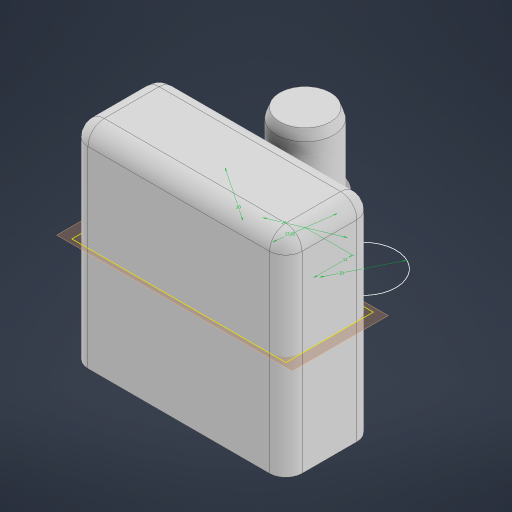
# Autodesk Inventor part: batteriehalter
Saved by Autodesk Inventor 2023 (Build 270158000, 158)
## iProperties
Created: 2023-05-28
Part Number: batteriehalter
Material: Generic
Document SubType Name: Modeling
Designer: bananenbrot
Density: 1 g/cm^3
Appearance: Default
Author: bananenbrot
Autodesk Inventor part; units mm, degrees
ref_plane "YZ Plane" through (0, 0, 0) normal (1, 0, 0) x (0, 1, 0)
ref_plane "XZ Plane" through (0, 0, 0) normal (0, 1, 0) x (-1, 0, 0)
ref_plane "XY Plane" through (0, 0, 0) normal (0, 0, 1) x (1, 0, 0)
sketch "Sketch1" plane through (0, 0, 0) normal (0, 1, 0) x (-1, 0, 0)
  line L0 (3.8011, 12.3974) -> (-62.0989, 12.3974)
  line L1 (-62.0989, 12.3974) -> (-62.0989, -14.5026)
  line L2 (-62.0989, -14.5026) -> (3.8011, -14.5026)
  line L3 (3.8011, -14.5026) -> (3.8011, 12.3974)
  line L4 (2.6011, 11.1974) -> (-60.8989, 11.1974)
  line L5 (-60.8989, 11.1974) -> (-60.8989, -13.3026)
  line L6 (-60.8989, -13.3026) -> (2.6011, -13.3026)
  line L7 (2.6011, -13.3026) -> (2.6011, 11.1974)
  point P0 (0, 0)
  dimension "d0" = 26.9
  dimension "d1" = 65.9
  dimension "d2" = 1.2
  dimension "d3" = 24.5
  dimension "d4" = 63.5
  constraints: 16 end point, 4 parallel, 2 perpendicular, 1 horizontal, 3 other
  measures "d0" distance of L2.end L0.start
  measures "d1" distance of L0.start L0.end
  measures "d2" distance between parallel lines of L3 L7
  measures "d3" distance of L6.end L4.start
  measures "d4" distance of L5.end L6.end
extrude "Extrusion1" add sketch "Sketch1" along normal blind 1.2 contours L3 L2 L1 L0 | L7 L6 L5 L4
extrude "Extrusion2" add sketch "Sketch1" against normal blind 63
fillet "Fillet1" radius 5 8 edges at (29.1489, 0, 11.1974) (-2.6011, -31.5, 11.1974) (-2.6011, 0, -1.0526) (29.1489, 0, -13.3026) (60.8989, 0, -1.0526) (60.8989, -31.5, -13.3026) (-2.6011, -31.5, -13.3026) (60.8989, -31.5, 11.1974)
ref_plane "Work Plane1" through (0, -30.9, 0) normal (0, 1, 0) x (1, 0, 0)
sketch "Sketch3" plane through (0, -30.9, 0) normal (0, 1, 0) x (1, 0, 0)
  arc A0 (2.3989, 13.3026) -> (-2.6011, 8.3026) centre (2.3989, 8.3026) ccw projected
  line L0 (-2.6011, 8.3026) -> (-2.6011, -6.1974) projected
  arc A1 (-2.6011, -6.1974) -> (2.3989, -11.1974) centre (2.3989, -6.1974) ccw projected
  line L1 (2.3989, -11.1974) -> (55.8989, -11.1974) projected
  arc A2 (55.8989, -11.1974) -> (60.8989, -6.1974) centre (55.8989, -6.1974) ccw projected
  line L2 (60.8989, -6.1974) -> (60.8989, 8.3026) projected
  arc A3 (60.8989, 8.3026) -> (55.8989, 13.3026) centre (55.8989, 8.3026) ccw projected
  line L3 (55.8989, 13.3026) -> (2.3989, 13.3026) projected
  line L4 (62.0989, -12.3974) -> (-3.8011, -12.3974) projected
  line L5 (-3.8011, -12.3974) -> (-3.8011, 14.5026) projected
  line L6 (-3.8011, 14.5026) -> (62.0989, 14.5026) projected
  line L7 (62.0989, 14.5026) -> (62.0989, -12.3974) projected
  circle A4 centre (29.1489, 26.5026) radius 8.825
  circle A5 centre (29.1489, 26.5026) radius 10
  circle A6 centre (9.2492, 24.5026) radius 10
  circle A7 centre (49.0487, 24.5026) radius 10
  point P0 (0, 0)
  point P1 (29.1489, 14.5026)
  point P2 (49.0487, 14.5026)
  point P3 (39.0988, 25.5026)
  point P4 (19.199, 25.5026)
  point P5 (9.2492, 14.5026)
  dimension "d10" = 17.65
  dimension "d11" = 20
  dimension "d12" = 12
  dimension "d13" = 20
  dimension "d14" = 20
  constraints: 4 centre point, 4 tangent, 1 coincident, 1 midpoint, 1 vertical alignment
  measures "d10" diameter of A4
  measures "d11" diameter of A5
  measures "d12" distance from line of A4.centre L6
  measures "d13" diameter of A6
  measures "d14" diameter of A7
extrude "Extrusion3" add sketch "Sketch3" along normal mid plane 20 contours L6 A6 A5 A7 | A5 | A4
extrude "Extrusion4" add sketch "Sketch3" along normal mid plane 64.2 contours A4
chamfer "Chamfer1" distance 1 distance2 3 1 edges at (20.3239, -63, -26.5026) measured on face at (20.8239, -63, -26.5026)
chamfer "Chamfer2" distance 1 distance2 3 1 edges at (20.3239, 1.2, -26.5026) measured on face at (20.8239, 1.2, -26.5026)
fillet "Fillet2" radius 5 8 edges at (62.0989, -30.9, -14.5026) (62.0989, -30.9, 12.3974) (-3.8011, -30.9, 12.3974) (-3.8011, -30.9, -14.5026) (-3.8011, 1.2, -1.0526) (29.1489, 1.2, 12.3974) (62.0989, 1.2, -1.0526) (29.1489, 1.2, -14.5026)
body "Solid1"
